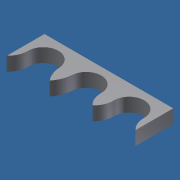
# Autodesk Inventor part: swirvy for illustrator
Saved by Autodesk Inventor 2012 (Build 160160000, 160)
## iProperties
Created: 2012-02-21
Part Number: swirvy for illustrator
Material: Default
Document SubType Name: Modeling
Designer: Allison Garza
Density: 1 g/cm^3
Author: Allison Garza
Autodesk Inventor part; units mm, degrees
ref_plane "YZ Plane" through (0, 0, 0) normal (1, 0, 0) x (0, 1, 0)
ref_plane "XZ Plane" through (0, 0, 0) normal (0, 1, 0) x (-1, 0, 0)
ref_plane "XY Plane" through (0, 0, 0) normal (0, 0, 1) x (1, 0, 0)
sketch "Sketch1" plane through (0, 0, 0) normal (0, 0, 1) x (1, 0, 0)
  line L0 (0, 0) -> (-476.25, 0)
  line L1 (-476.25, 0) -> (-476.25, 50.8)
  line L2 (-476.25, 50.8) -> (0, 50.8)
  line L3 (0, 50.8) -> (0, 0)
  dimension "d5" = 50.8
  dimension "d6" = 476.25
  constraints: 8 end point, 2 parallel, 1 horizontal, 1 perpendicular
  measures "d5" distance of L2.end L0.start
  measures "d6" distance of L0.start L0.end
extrude "Extrusion1" add sketch "Sketch1" against normal blind 139.7
sketch "Sketch2" plane through (-476.25, 50.8, 0) normal (0, 1, 0) x (1, 0, 0)
  line L0 (0, 0) -> (476.25, 0) projected
  circle A0 centre (396.875, 55.88) radius 55.88
  arc A1 (452.7532, 55.4333) -> (476.25, 0) centre (528.4627, 54.8281) ccw
  line L1 (476.25, 139.7) -> (0, 139.7) projected
  line L2 (476.25, 0) -> (476.25, 139.7) projected
  line L3 (158.75, 139.7) -> (158.75, 0)
  line L4 (317.5, 139.7) -> (317.5, 0)
  circle A2 centre (238.125, 55.88) radius 55.88
  circle A3 centre (79.375, 55.88) radius 55.88
  arc A4 (317.5, 0) -> (341.0467, 58.2841) centre (268.3126, 53.7701) ccw
  arc A5 (135.1205, 59.7553) -> (158.75, 0) centre (241.1273, 67.1248) ccw
  arc A6 (0, 0) -> (23.4968, 55.4333) centre (-52.2127, 54.8281) ccw
  arc A7 (158.75, 0) -> (182.3795, 59.7553) centre (76.3727, 67.1248) ccw
  arc A8 (293.9963, 54.8959) -> (317.5, 0) centre (366.8591, 53.6126) ccw
  dimension "d9" = 111.76
  dimension "d10" = 55.88
  dimension "d11" = 79.375
  dimension "d14" = 158.75
  dimension "d15" = 158.75
  dimension "d16" = 79.375
  dimension "d17" = 79.375
  constraints: 18 point on circle, 9 centre point, 7 tangent, 4 end point, 4 point on line, 3 equal radius, 2 perpendicular
  measures "d9" diameter of A0
  measures "d10" vertical distance of L0.end A0.centre
  measures "d11" horizontal distance of L0.end A0.centre
  measures "d14" distance between parallel lines of L2 L4
  measures "d15" distance between parallel lines of L4 L3
  measures "d16" horizontal distance of L1.end A3.centre
  measures "d17" horizontal distance of L3.start A2.centre
extrude "Extrusion3" cut sketch "Sketch2" against normal blind 139.7 contours A6 A3 L0 | A7 A2 L0 | A3 A5 L0 | A3 | A2 A8 L0 | A2 | A4 A0 L0 | A0 A1 L0 | A0 A4 picked at (415.2449, 59.3205)
body "Solid1"
